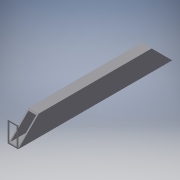
# Autodesk Inventor part: lift brace
Saved by Autodesk Inventor 2018 (Build 220112000, 112)
## iProperties
Created: 2018-02-04
Part Number: lift brace
Material: Generic
Document SubType Name: Modeling
Designer: Luke
Density: 1 g/cm^3
Appearance: Default
Author: Luke
Autodesk Inventor part; units mm, degrees
ref_plane "YZ Plane" through (0, 0, 0) normal (1, 0, 0) x (0, 1, 0)
ref_plane "XZ Plane" through (0, 0, 0) normal (0, 1, 0) x (-1, 0, 0)
ref_plane "XY Plane" through (0, 0, 0) normal (0, 0, 1) x (1, 0, 0)
sketch "Sketch1" plane through (0, 0, 0) normal (0, 0, 1) x (1, 0, 0)
  line L0 (0, 0) -> (25.4, 0)
  line L1 (25.4, 0) -> (25.4, 50.8)
  line L2 (25.4, 50.8) -> (0, 50.8)
  line L3 (0, 50.8) -> (0, 0)
  line L4 (3.175, 47.625) -> (22.225, 47.625)
  line L5 (22.225, 47.625) -> (22.225, 3.175)
  line L6 (22.225, 3.175) -> (3.175, 3.175)
  line L7 (3.175, 3.175) -> (3.175, 47.625)
  dimension "d0" = 25.4
  dimension "d1" = 50.8
  dimension "d2" = 3.175
  constraints: 16 end point, 4 parallel, 2 perpendicular, 1 horizontal, 3 other
  measures "d0" distance of L2.end L1.end
  measures "d1" distance of L1.end L0.end
  measures "d2" distance between parallel lines of L2 L4
extrude "Extrusion1" add sketch "Sketch1" along normal blind 381
sketch "Sketch2" plane through (25.4, 0, 0) normal (1, 0, 0) x (0, 0, -1)
  line L0 (-25.4, 50.8) -> (0, 50.8)
  line L1 (0, 50.8) -> (0, 0)
  line L2 (0, 0) -> (-25.4, 50.8)
  line L3 (0, 50.8) -> (-381, 50.8) projected
  line L4 (-381, 50.8) -> (-381, 0)
  line L5 (-381, 50.8) -> (-254, 50.8)
  line L6 (-381, 0) -> (-353.6689, 0)
  line L7 (-353.6689, 0) -> (-379.0689, 0)
  line L8 (-353.6689, 0) -> (-254, 50.8)
  point P0 (-329.9529, 50.8)
  point P1 (-355.3529, 88.9)
  dimension "d8" = 50.8
  dimension "d9" = 25.4
  dimension "d16" = 50.8
  dimension "d17" = 127
  dimension "d18" = 25.4
  constraints: 16 end point, 1 horizontal, 1 perpendicular, 1 point on line, 1 vertical, 2 other
  measures "d8" distance of L0.end L1.end
  measures "d9" distance of L0.start L0.end
  measures "d16" distance of L4.end L4.start
  measures "d17" distance of L4.start L5.end
  measures "d18" distance of L6.end L7.end
extrude "Extrusion2" cut sketch "Sketch2" against normal blind 381
body "Solid1"
